Autodesk Fusion 360 part; units mm, degrees
(part 3 of 5)
  spline S77 degree 5 poles (-23.4359, 13.9427) (-23.4388, 13.9438) (-23.4499, 13.948) (-23.4693, 13.9553) (-23.4971, 13.9654) (-23.5331, 13.9784) (-23.5747, 13.9929) (-23.6165, 14.0072) (-23.6584, 14.0212) (-23.7004, 14.0348) (-23.7426, 14.0482) (-23.7849, 14.0612) (-23.8274, 14.074) (-23.87, 14.0865) (-23.9128, 14.0988) (-23.9556, 14.1108) (-23.9986, 14.1225) (-24.0417, 14.134) (-24.0849, 14.1453) (-24.1282, 14.1563) (-24.1716, 14.1671) (-24.2152, 14.1777) (-24.2588, 14.188) (-24.3025, 14.1981) (-24.3464, 14.208) (-24.3903, 14.2176) (-24.4343, 14.2271) (-24.4785, 14.2363) (-24.5227, 14.2453) (-24.567, 14.2541) (-24.6114, 14.2627) (-24.6559, 14.2711) (-24.7005, 14.2793) (-24.7451, 14.2873) (-24.7899, 14.2951) (-24.8347, 14.3027) (-24.8796, 14.3101) (-24.9246, 14.3173) (-24.9697, 14.3243) (-25.0148, 14.3311) (-25.06, 14.3377) (-25.1053, 14.3442) (-25.1507, 14.3504) (-25.1962, 14.3565) (-25.2417, 14.3624) (-25.2873, 14.3681) (-25.3329, 14.3736) (-25.3786, 14.3789) (-25.4244, 14.3841) (-25.4703, 14.3891) (-25.5162, 14.3939) (-25.5622, 14.3985) (-25.6082, 14.4029) (-25.6544, 14.4072) (-25.7005, 14.4113) (-25.7468, 14.4152) (-25.7931, 14.419) (-25.8395, 14.4226) (-25.8859, 14.426) (-25.9324, 14.4293) (-25.9789, 14.4323) (-26.0255, 14.4352) (-26.0628, 14.4374) (-26.0908, 14.439) (-26.1095, 14.44) (-26.1189, 14.4405) knots 0.13777296 0.13777296 0.13777296 0.13777296 0.13777296 0.13777296 0.14285714 0.15714286 0.17142857 0.18571429 0.2 0.21428571 0.22857143 0.24285714 0.25714286 0.27142857 0.28571429 0.3 0.31428571 0.32857143 0.34285714 0.35714286 0.37142857 0.38571429 0.4 0.41428571 0.42857143 0.44285714 0.45714286 0.47142857 0.48571429 0.5 0.51428571 0.52857143 0.54285714 0.55714286 0.57142857 0.58571429 0.6 0.61428571 0.62857143 0.64285714 0.65714286 0.67142857 0.68571429 0.7 0.71428571 0.72857143 0.74285714 0.75714286 0.77142857 0.78571429 0.8 0.81428571 0.82857143 0.84285714 0.85714286 0.87142857 0.88571429 0.9 0.91428571 0.92857143 0.94285714 0.95714286 0.97142857 0.98571429 1 1 1 1 1 1
  arc A39 (-26.1189, 14.4405) -> (-26.5772, 13.5785) centre (0, 0) ccw
  spline S78 degree 5 poles (-26.5772, 13.5785) (-26.5716, 13.571) (-26.5603, 13.5561) (-26.5433, 13.5337) (-26.5206, 13.504) (-26.4922, 13.467) (-26.4636, 13.4302) (-26.4349, 13.3934) (-26.4061, 13.3569) (-26.3772, 13.3204) (-26.3482, 13.2842) (-26.3191, 13.248) (-26.2899, 13.212) (-26.2605, 13.1762) (-26.2311, 13.1405) (-26.2015, 13.1049) (-26.1719, 13.0696) (-26.1421, 13.0343) (-26.1122, 12.9992) (-26.0822, 12.9643) (-26.0521, 12.9296) (-26.0219, 12.895) (-25.9916, 12.8605) (-25.9611, 12.8262) (-25.9306, 12.7921) (-25.8999, 12.7582) (-25.8691, 12.7244) (-25.8382, 12.6908) (-25.8072, 12.6573) (-25.7761, 12.6241) (-25.7448, 12.591) (-25.7135, 12.558) (-25.682, 12.5253) (-25.6504, 12.4927) (-25.6187, 12.4604) (-25.5868, 12.4282) (-25.5549, 12.3962) (-25.5228, 12.3644) (-25.4906, 12.3327) (-25.4583, 12.3013) (-25.4258, 12.2701) (-25.3933, 12.2391) (-25.3605, 12.2082) (-25.3277, 12.1776) (-25.2948, 12.1472) (-25.2617, 12.117) (-25.2284, 12.0871) (-25.1951, 12.0573) (-25.1616, 12.0278) (-25.1279, 11.9985) (-25.0942, 11.9695) (-25.0603, 11.9407) (-25.0262, 11.9121) (-24.992, 11.8837) (-24.9576, 11.8557) (-24.9231, 11.8279) (-24.8885, 11.8004) (-24.8537, 11.7731) (-24.8187, 11.7462) (-24.7835, 11.7196) (-24.7482, 11.6933) (-24.7172, 11.6706) (-24.6933, 11.6533) (-24.6765, 11.6412) (-24.6668, 11.6343) (-24.6642, 11.6325) knots -1 -1 -1 -1 -1 -1 -0.98571429 -0.97142857 -0.95714286 -0.94285714 -0.92857143 -0.91428571 -0.9 -0.88571429 -0.87142857 -0.85714286 -0.84285714 -0.82857143 -0.81428571 -0.8 -0.78571429 -0.77142857 -0.75714286 -0.74285714 -0.72857143 -0.71428571 -0.7 -0.68571429 -0.67142857 -0.65714286 -0.64285714 -0.62857143 -0.61428571 -0.6 -0.58571429 -0.57142857 -0.55714286 -0.54285714 -0.52857143 -0.51428571 -0.5 -0.48571429 -0.47142857 -0.45714286 -0.44285714 -0.42857143 -0.41428571 -0.4 -0.38571429 -0.37142857 -0.35714286 -0.34285714 -0.32857143 -0.31428571 -0.3 -0.28571429 -0.27142857 -0.25714286 -0.24285714 -0.22857143 -0.21428571 -0.2 -0.18571429 -0.17142857 -0.15714286 -0.14285714 -0.13777296 -0.13777296 -0.13777296 -0.13777296 -0.13777296 -0.13777296
  spline S79 degree 3 poles (-24.5985, 11.3854) (-24.5876, 11.4091) (-24.5813, 11.4346) (-24.579, 11.4866) (-24.583, 11.5126) (-24.5987, 11.5563) (-24.6084, 11.5742) (-24.633, 11.6066) (-24.6477, 11.6208) (-24.6642, 11.6325) knots 0 0 0 0 0.007813 0.007813 0.015626 0.015626 0.021719 0.021719 0.027811 0.027811 0.027811 0.027811
  arc A40 (-24.5985, 11.3854) -> (-24.9206, 10.6619) centre (0, 0) ccw
  spline S80 degree 3 poles (-25.1482, 10.5454) (-25.1228, 10.5397) (-25.0965, 10.539) (-25.0452, 10.5478) (-25.0206, 10.5572) (-24.9813, 10.5817) (-24.9658, 10.595) (-24.9394, 10.6259) (-24.9286, 10.6432) (-24.9206, 10.6619) knots 0 0 0 0 0.007813 0.007813 0.015626 0.015626 0.021719 0.021719 0.027811 0.027811 0.027811 0.027811
  spline S81 degree 5 poles (-25.1482, 10.5454) (-25.1513, 10.5461) (-25.1629, 10.5487) (-25.1831, 10.5531) (-25.212, 10.5594) (-25.2495, 10.5672) (-25.2927, 10.5758) (-25.3361, 10.5841) (-25.3795, 10.5921) (-25.423, 10.5998) (-25.4667, 10.6071) (-25.5104, 10.6141) (-25.5543, 10.6209) (-25.5982, 10.6274) (-25.6422, 10.6335) (-25.6863, 10.6395) (-25.7305, 10.6451) (-25.7748, 10.6505) (-25.8191, 10.6557) (-25.8636, 10.6606) (-25.9081, 10.6652) (-25.9526, 10.6696) (-25.9973, 10.6737) (-26.042, 10.6776) (-26.0868, 10.6813) (-26.1317, 10.6848) (-26.1766, 10.688) (-26.2216, 10.691) (-26.2666, 10.6938) (-26.3117, 10.6963) (-26.3569, 10.6987) (-26.4021, 10.7008) (-26.4474, 10.7027) (-26.4927, 10.7044) (-26.5381, 10.7059) (-26.5836, 10.7071) (-26.6291, 10.7082) (-26.6746, 10.7091) (-26.7202, 10.7098) (-26.7659, 10.7102) (-26.8116, 10.7105) (-26.8573, 10.7106) (-26.9031, 10.7105) (-26.949, 10.7101) (-26.9949, 10.7096) (-27.0408, 10.7089) (-27.0868, 10.708) (-27.1328, 10.707) (-27.1789, 10.7057) (-27.225, 10.7042) (-27.2711, 10.7026) (-27.3173, 10.7008) (-27.3635, 10.6988) (-27.4098, 10.6966) (-27.4561, 10.6942) (-27.5024, 10.6917) (-27.5488, 10.689) (-27.5952, 10.6861) (-27.6417, 10.683) (-27.6882, 10.6797) (-27.7347, 10.6763) (-27.7812, 10.6727) (-27.8185, 10.6697) (-27.8464, 10.6673) (-27.8651, 10.6658) (-27.8744, 10.6649) knots 0.13777296 0.13777296 0.13777296 0.13777296 0.13777296 0.13777296 0.14285714 0.15714286 0.17142857 0.18571429 0.2 0.21428571 0.22857143 0.24285714 0.25714286 0.27142857 0.28571429 0.3 0.31428571 0.32857143 0.34285714 0.35714286 0.37142857 0.38571429 0.4 0.41428571 0.42857143 0.44285714 0.45714286 0.47142857 0.48571429 0.5 0.51428571 0.52857143 0.54285714 0.55714286 0.57142857 0.58571429 0.6 0.61428571 0.62857143 0.64285714 0.65714286 0.67142857 0.68571429 0.7 0.71428571 0.72857143 0.74285714 0.75714286 0.77142857 0.78571429 0.8 0.81428571 0.82857143 0.84285714 0.85714286 0.87142857 0.88571429 0.9 0.91428571 0.92857143 0.94285714 0.95714286 0.97142857 0.98571429 1 1 1 1 1 1
  arc A41 (-27.8744, 10.6649) -> (-28.2083, 9.7475) centre (0, 0) ccw
  spline S82 degree 5 poles (-28.2083, 9.7475) (-28.2017, 9.7409) (-28.1884, 9.7277) (-28.1685, 9.7079) (-28.1419, 9.6816) (-28.1086, 9.649) (-28.0752, 9.6164) (-28.0416, 9.5841) (-28.008, 9.5519) (-27.9744, 9.5198) (-27.9406, 9.4879) (-27.9067, 9.4562) (-27.8728, 9.4246) (-27.8387, 9.3932) (-27.8046, 9.3619) (-27.7704, 9.3309) (-27.7361, 9.2999) (-27.7017, 9.2692) (-27.6672, 9.2386) (-27.6327, 9.2082) (-27.598, 9.178) (-27.5633, 9.1479) (-27.5285, 9.118) (-27.4935, 9.0883) (-27.4585, 9.0588) (-27.4234, 9.0294) (-27.3883, 9.0003) (-27.353, 8.9713) (-27.3176, 8.9425) (-27.2822, 8.9139) (-27.2466, 8.8854) (-27.211, 8.8572) (-27.1753, 8.8292) (-27.1394, 8.8013) (-27.1035, 8.7737) (-27.0675, 8.7462) (-27.0314, 8.719) (-26.9952, 8.6919) (-26.9589, 8.6651) (-26.9225, 8.6385) (-26.8861, 8.6121) (-26.8495, 8.5859) (-26.8128, 8.5599) (-26.776, 8.5342) (-26.7392, 8.5087) (-26.7022, 8.4834) (-26.6651, 8.4583) (-26.6279, 8.4335) (-26.5907, 8.4089) (-26.5533, 8.3846) (-26.5158, 8.3605) (-26.4782, 8.3367) (-26.4405, 8.3132) (-26.4027, 8.2899) (-26.3648, 8.2669) (-26.3267, 8.2441) (-26.2886, 8.2217) (-26.2503, 8.1996) (-26.2119, 8.1778) (-26.1734, 8.1563) (-26.1347, 8.1352) (-26.1009, 8.117) (-26.0748, 8.1032) (-26.0565, 8.0936) (-26.0459, 8.0882) (-26.0431, 8.0867) knots -1 -1 -1 -1 -1 -1 -0.98571429 -0.97142857 -0.95714286 -0.94285714 -0.92857143 -0.91428571 -0.9 -0.88571429 -0.87142857 -0.85714286 -0.84285714 -0.82857143 -0.81428571 -0.8 -0.78571429 -0.77142857 -0.75714286 -0.74285714 -0.72857143 -0.71428571 -0.7 -0.68571429 -0.67142857 -0.65714286 -0.64285714 -0.62857143 -0.61428571 -0.6 -0.58571429 -0.57142857 -0.55714286 -0.54285714 -0.52857143 -0.51428571 -0.5 -0.48571429 -0.47142857 -0.45714286 -0.44285714 -0.42857143 -0.41428571 -0.4 -0.38571429 -0.37142857 -0.35714286 -0.34285714 -0.32857143 -0.31428571 -0.3 -0.28571429 -0.27142857 -0.25714286 -0.24285714 -0.22857143 -0.21428571 -0.2 -0.18571429 -0.17142857 -0.15714286 -0.14285714 -0.13777296 -0.13777296 -0.13777296 -0.13777296 -0.13777296 -0.13777296
  spline S83 degree 3 poles (-25.9437, 7.8512) (-25.9361, 7.8761) (-25.9335, 7.9023) (-25.9385, 7.9541) (-25.946, 7.9793) (-25.9676, 8.0203) (-25.9798, 8.0367) (-26.0086, 8.0653) (-26.0251, 8.0774) (-26.0431, 8.0867) knots 0 0 0 0 0.007813 0.007813 0.015626 0.015626 0.021719 0.021719 0.027811 0.027811 0.027811 0.027811
  arc A42 (-25.9437, 7.8512) -> (-26.162, 7.0899) centre (0, 0) ccw
  spline S84 degree 3 poles (-26.3711, 6.9428) (-26.3452, 6.9407) (-26.3191, 6.9437) (-26.2694, 6.9595) (-26.2464, 6.9722) (-26.2109, 7.002) (-26.1974, 7.0174) (-26.1755, 7.0516) (-26.1673, 7.0703) (-26.162, 7.0899) knots 0 0 0 0 0.007813 0.007813 0.015626 0.015626 0.021719 0.021719 0.027811 0.027811 0.027811 0.027811
  spline S85 degree 5 poles (-26.3711, 6.9428) (-26.3742, 6.9431) (-26.3861, 6.944) (-26.4068, 6.9456) (-26.4362, 6.9478) (-26.4745, 6.9503) (-26.5185, 6.9528) (-26.5625, 6.955) (-26.6066, 6.9569) (-26.6508, 6.9584) (-26.695, 6.9596) (-26.7393, 6.9605) (-26.7837, 6.9611) (-26.8281, 6.9613) (-26.8726, 6.9613) (-26.9171, 6.9611) (-26.9616, 6.9605) (-27.0062, 6.9597) (-27.0508, 6.9586) (-27.0955, 6.9573) (-27.1402, 6.9557) (-27.185, 6.9538) (-27.2298, 6.9517) (-27.2746, 6.9494) (-27.3195, 6.9468) (-27.3644, 6.944) (-27.4093, 6.9409) (-27.4543, 6.9376) (-27.4993, 6.9341) (-27.5443, 6.9303) (-27.5893, 6.9264) (-27.6344, 6.9222) (-27.6795, 6.9178) (-27.7247, 6.9131) (-27.7698, 6.9083) (-27.815, 6.9032) (-27.8602, 6.898) (-27.9054, 6.8925) (-27.9507, 6.8868) (-27.996, 6.8809) (-28.0413, 6.8748) (-28.0866, 6.8685) (-28.1319, 6.862) (-28.1773, 6.8553) (-28.2227, 6.8484) (-28.268, 6.8414) (-28.3135, 6.8341) (-28.3589, 6.8266) (-28.4043, 6.8189) (-28.4498, 6.8111) (-28.4952, 6.803) (-28.5407, 6.7948) (-28.5862, 6.7864) (-28.6317, 6.7778) (-28.6772, 6.769) (-28.7228, 6.76) (-28.7683, 6.7509) (-28.8139, 6.7416) (-28.8594, 6.732) (-28.905, 6.7224) (-28.9506, 6.7125) (-28.9962, 6.7024) (-29.0327, 6.6943) (-29.06, 6.6881) (-29.0783, 6.6839) (-29.0874, 6.6818) knots 0.13777296 0.13777296 0.13777296 0.13777296 0.13777296 0.13777296 0.14285714 0.15714286 0.17142857 0.18571429 0.2 0.21428571 0.22857143 0.24285714 0.25714286 0.27142857 0.28571429 0.3 0.31428571 0.32857143 0.34285714 0.35714286 0.37142857 0.38571429 0.4 0.41428571 0.42857143 0.44285714 0.45714286 0.47142857 0.48571429 0.5 0.51428571 0.52857143 0.54285714 0.55714286 0.57142857 0.58571429 0.6 0.61428571 0.62857143 0.64285714 0.65714286 0.67142857 0.68571429 0.7 0.71428571 0.72857143 0.74285714 0.75714286 0.77142857 0.78571429 0.8 0.81428571 0.82857143 0.84285714 0.85714286 0.87142857 0.88571429 0.9 0.91428571 0.92857143 0.94285714 0.95714286 0.97142857 0.98571429 1 1 1 1 1 1
  arc A43 (-29.0874, 6.6818) -> (-29.2904, 5.7268) centre (0, 0) ccw
  spline S86 degree 5 poles (-29.2904, 5.7268) (-29.2829, 5.7212) (-29.268, 5.7099) (-29.2455, 5.6931) (-29.2155, 5.6708) (-29.1779, 5.6431) (-29.1403, 5.6156) (-29.1026, 5.5882) (-29.0648, 5.5609) (-29.027, 5.5339) (-28.9891, 5.507) (-28.9512, 5.4803) (-28.9132, 5.4537) (-28.8751, 5.4274) (-28.8369, 5.4012) (-28.7987, 5.3752) (-28.7605, 5.3493) (-28.7221, 5.3237) (-28.6838, 5.2982) (-28.6453, 5.2729) (-28.6068, 5.2478) (-28.5682, 5.2228) (-28.5295, 5.1981) (-28.4908, 5.1735) (-28.4521, 5.1491) (-28.4132, 5.125) (-28.3743, 5.101) (-28.3353, 5.0772) (-28.2963, 5.0536) (-28.2572, 5.0302) (-28.2181, 5.007) (-28.1789, 4.984) (-28.1396, 4.9612) (-28.1002, 4.9386) (-28.0608, 4.9162) (-28.0213, 4.894) (-27.9818, 4.8721) (-27.9422, 4.8503) (-27.9025, 4.8288) (-27.8628, 4.8075) (-27.823, 4.7865) (-27.7831, 4.7656) (-27.7432, 4.745) (-27.7032, 4.7246) (-27.6631, 4.7045) (-27.623, 4.6846) (-27.5828, 4.6649) (-27.5425, 4.6455) (-27.5022, 4.6264) (-27.4618, 4.6075) (-27.4213, 4.5889) (-27.3807, 4.5705) (-27.3401, 4.5525) (-27.2995, 4.5347) (-27.2587, 4.5171) (-27.2179, 4.4999) (-27.177, 4.483) (-27.136, 4.4665) (-27.0949, 4.4502) (-27.0538, 4.4343) (-27.0126, 4.4188) (-26.9766, 4.4055) (-26.9488, 4.3955) (-26.9293, 4.3885) (-26.9181, 4.3846) (-26.9151, 4.3835) knots -1 -1 -1 -1 -1 -1 -0.98571429 -0.97142857 -0.95714286 -0.94285714 -0.92857143 -0.91428571 -0.9 -0.88571429 -0.87142857 -0.85714286 -0.84285714 -0.82857143 -0.81428571 -0.8 -0.78571429 -0.77142857 -0.75714286 -0.74285714 -0.72857143 -0.71428571 -0.7 -0.68571429 -0.67142857 -0.65714286 -0.64285714 -0.62857143 -0.61428571 -0.6 -0.58571429 -0.57142857 -0.55714286 -0.54285714 -0.52857143 -0.51428571 -0.5 -0.48571429 -0.47142857 -0.45714286 -0.44285714 -0.42857143 -0.41428571 -0.4 -0.38571429 -0.37142857 -0.35714286 -0.34285714 -0.32857143 -0.31428571 -0.3 -0.28571429 -0.27142857 -0.25714286 -0.24285714 -0.22857143 -0.21428571 -0.2 -0.18571429 -0.17142857 -0.15714286 -0.14285714 -0.13777296 -0.13777296 -0.13777296 -0.13777296 -0.13777296 -0.13777296
  spline S87 degree 3 poles (-26.7838, 4.1641) (-26.7798, 4.1898) (-26.7809, 4.2161) (-26.793, 4.2668) (-26.804, 4.2907) (-26.8311, 4.3283) (-26.8454, 4.3428) (-26.878, 4.3672) (-26.896, 4.3768) (-26.9151, 4.3835) knots 0 0 0 0 0.007813 0.007813 0.015626 0.015626 0.021719 0.021719 0.027811 0.027811 0.027811 0.027811
  arc A44 (-26.7838, 4.1641) -> (-26.8941, 3.3798) centre (0, 0) ccw
  spline S88 degree 3 poles (-27.0807, 3.2051) (-27.0547, 3.2066) (-27.0293, 3.2132) (-26.9824, 3.2358) (-26.9613, 3.2516) (-26.9303, 3.286) (-26.9191, 3.3031) (-26.9022, 3.34) (-26.8966, 3.3597) (-26.8941, 3.3798) knots 0 0 0 0 0.007813 0.007813 0.015626 0.015626 0.021719 0.021719 0.027811 0.027811 0.027811 0.027811
  spline S89 degree 5 poles (-27.0807, 3.2051) (-27.0839, 3.2049) (-27.0958, 3.2042) (-27.1164, 3.2029) (-27.1459, 3.2009) (-27.1841, 3.1981) (-27.228, 3.1945) (-27.272, 3.1905) (-27.3159, 3.1862) (-27.3599, 3.1816) (-27.4038, 3.1766) (-27.4478, 3.1714) (-27.4918, 3.1657) (-27.5359, 3.1599) (-27.5799, 3.1537) (-27.6239, 3.1472) (-27.6679, 3.1405) (-27.712, 3.1334) (-27.756, 3.1262) (-27.8001, 3.1186) (-27.8442, 3.1108) (-27.8882, 3.1027) (-27.9323, 3.0944) (-27.9763, 3.0859) (-28.0204, 3.0771) (-28.0645, 3.068) (-28.1086, 3.0587) (-28.1526, 3.0492) (-28.1967, 3.0395) (-28.2407, 3.0295) (-28.2848, 3.0193) (-28.3289, 3.0088) (-28.3729, 2.9982) (-28.417, 2.9873) (-28.461, 2.9762) (-28.5051, 2.9649) (-28.5491, 2.9534) (-28.5931, 2.9417) (-28.6371, 2.9298) (-28.6812, 2.9177) (-28.7252, 2.9053) (-28.7692, 2.8928) (-28.8132, 2.88) (-28.8571, 2.8671) (-28.9011, 2.854) (-28.9451, 2.8406) (-28.989, 2.8271) (-29.033, 2.8134) (-29.0769, 2.7995) (-29.1208, 2.7854) (-29.1647, 2.7711) (-29.2086, 2.7566) (-29.2525, 2.7419) (-29.2964, 2.7271) (-29.3402, 2.712) (-29.3841, 2.6968) (-29.4279, 2.6814) (-29.4717, 2.6658) (-29.5155, 2.6501) (-29.5593, 2.6341) (-29.6031, 2.618) (-29.6468, 2.6017) (-29.6818, 2.5886) (-29.708, 2.5786) (-29.7255, 2.5719) (-29.7343, 2.5686) knots 0.13777296 0.13777296 0.13777296 0.13777296 0.13777296 0.13777296 0.14285714 0.15714286 0.17142857 0.18571429 0.2 0.21428571 0.22857143 0.24285714 0.25714286 0.27142857 0.28571429 0.3 0.31428571 0.32857143 0.34285714 0.35714286 0.37142857 0.38571429 0.4 0.41428571 0.42857143 0.44285714 0.45714286 0.47142857 0.48571429 0.5 0.51428571 0.52857143 0.54285714 0.55714286 0.57142857 0.58571429 0.6 0.61428571 0.62857143 0.64285714 0.65714286 0.67142857 0.68571429 0.7 0.71428571 0.72857143 0.74285714 0.75714286 0.77142857 0.78571429 0.8 0.81428571 0.82857143 0.84285714 0.85714286 0.87142857 0.88571429 0.9 0.91428571 0.92857143 0.94285714 0.95714286 0.97142857 0.98571429 1 1 1 1 1 1
  arc A45 (-29.7343, 2.5686) -> (-29.8024, 1.5946) centre (0, 0) ccw
  spline S90 degree 5 poles (-29.8024, 1.5946) (-29.7942, 1.5901) (-29.7778, 1.5811) (-29.7532, 1.5675) (-29.7204, 1.5496) (-29.6793, 1.5274) (-29.6382, 1.5054) (-29.5971, 1.4835) (-29.5559, 1.4618) (-29.5147, 1.4403) (-29.4734, 1.4189) (-29.4321, 1.3977) (-29.3908, 1.3767) (-29.3494, 1.3559) (-29.308, 1.3353) (-29.2666, 1.3148) (-29.2251, 1.2946) (-29.1835, 1.2745) (-29.142, 1.2546) (-29.1004, 1.2349) (-29.0587, 1.2154) (-29.017, 1.1961) (-28.9753, 1.1769) (-28.9336, 1.158) (-28.8918, 1.1393) (-28.85, 1.1207) (-28.8081, 1.1024) (-28.7662, 1.0842) (-28.7243, 1.0663) (-28.6823, 1.0486) (-28.6403, 1.031) (-28.5983, 1.0137) (-28.5562, 0.9966) (-28.5141, 0.9797) (-28.4719, 0.9631) (-28.4297, 0.9466) (-28.3875, 0.9304) (-28.3453, 0.9143) (-28.303, 0.8986) (-28.2607, 0.883) (-28.2183, 0.8677) (-28.176, 0.8526) (-28.1336, 0.8377) (-28.0911, 0.8231) (-28.0486, 0.8087) (-28.0061, 0.7946) (-27.9636, 0.7808) (-27.921, 0.7672) (-27.8784, 0.7538) (-27.8358, 0.7407) (-27.7931, 0.7279) (-27.7504, 0.7154) (-27.7076, 0.7032) (-27.6649, 0.6912) (-27.6221, 0.6795) (-27.5793, 0.6681) (-27.5364, 0.6571) (-27.4935, 0.6464) (-27.4506, 0.636) (-27.4076, 0.626) (-27.3647, 0.6163) (-27.3272, 0.6082) (-27.2983, 0.6021) (-27.278, 0.598) (-27.2663, 0.5956) (-27.2633, 0.595) knots -1 -1 -1 -1 -1 -1 -0.98571429 -0.97142857 -0.95714286 -0.94285714 -0.92857143 -0.91428571 -0.9 -0.88571429 -0.87142857 -0.85714286 -0.84285714 -0.82857143 -0.81428571 -0.8 -0.78571429 -0.77142857 -0.75714286 -0.74285714 -0.72857143 -0.71428571 -0.7 -0.68571429 -0.67142857 -0.65714286 -0.64285714 -0.62857143 -0.61428571 -0.6 -0.58571429 -0.57142857 -0.55714286 -0.54285714 -0.52857143 -0.51428571 -0.5 -0.48571429 -0.47142857 -0.45714286 -0.44285714 -0.42857143 -0.41428571 -0.4 -0.38571429 -0.37142857 -0.35714286 -0.34285714 -0.32857143 -0.31428571 -0.3 -0.28571429 -0.27142857 -0.25714286 -0.24285714 -0.22857143 -0.21428571 -0.2 -0.18571429 -0.17142857 -0.15714286 -0.14285714 -0.13777296 -0.13777296 -0.13777296 -0.13777296 -0.13777296 -0.13777296
  spline S91 degree 3 poles (-27.1027, 0.396) (-27.1023, 0.422) (-27.107, 0.4479) (-27.1261, 0.4964) (-27.1403, 0.5185) (-27.1724, 0.552) (-27.1886, 0.5644) (-27.2242, 0.584) (-27.2434, 0.591) (-27.2633, 0.595) knots 0 0 0 0 0.007813 0.007813 0.015626 0.015626 0.021719 0.021719 0.027811 0.027811 0.027811 0.027811
  arc A46 (-27.1027, 0.396) -> (-27.1027, -0.396) centre (0, 0) ccw
  spline S92 degree 3 poles (-27.2633, -0.595) (-27.2377, -0.5899) (-27.2134, -0.5798) (-27.1701, -0.5509) (-27.1515, -0.5324) (-27.1255, -0.4939) (-27.1168, -0.4755) (-27.1052, -0.4365) (-27.1024, -0.4163) (-27.1027, -0.396) knots 0 0 0 0 0.007813 0.007813 0.015626 0.015626 0.021719 0.021719 0.027811 0.027811 0.027811 0.027811
  spline S93 degree 5 poles (-27.2633, -0.595) (-27.2663, -0.5956) (-27.278, -0.598) (-27.2983, -0.6021) (-27.3272, -0.6082) (-27.3647, -0.6163) (-27.4076, -0.626) (-27.4506, -0.636) (-27.4935, -0.6464) (-27.5364, -0.6571) (-27.5793, -0.6681) (-27.6221, -0.6795) (-27.6649, -0.6912) (-27.7076, -0.7032) (-27.7504, -0.7154) (-27.7931, -0.7279) (-27.8358, -0.7407) (-27.8784, -0.7538) (-27.921, -0.7672) (-27.9636, -0.7808) (-28.0061, -0.7946) (-28.0486, -0.8087) (-28.0911, -0.8231) (-28.1336, -0.8377) (-28.176, -0.8526) (-28.2183, -0.8677) (-28.2607, -0.883) (-28.303, -0.8986) (-28.3453, -0.9143) (-28.3875, -0.9304) (-28.4297, -0.9466) (-28.4719, -0.9631) (-28.5141, -0.9797) (-28.5562, -0.9966) (-28.5983, -1.0137) (-28.6403, -1.031) (-28.6823, -1.0486) (-28.7243, -1.0663) (-28.7662, -1.0842) (-28.8081, -1.1024) (-28.85, -1.1207) (-28.8918, -1.1393) (-28.9336, -1.158) (-28.9753, -1.1769) (-29.017, -1.1961) (-29.0587, -1.2154) (-29.1004, -1.2349) (-29.142, -1.2546) (-29.1835, -1.2745) (-29.2251, -1.2946) (-29.2666, -1.3148) (-29.308, -1.3353) (-29.3494, -1.3559) (-29.3908, -1.3767) (-29.4321, -1.3977) (-29.4734, -1.4189) (-29.5147, -1.4403) (-29.5559, -1.4618) (-29.5971, -1.4835) (-29.6382, -1.5054) (-29.6793, -1.5274) (-29.7204, -1.5496) (-29.7532, -1.5675) (-29.7778, -1.5811) (-29.7942, -1.5901) (-29.8024, -1.5946) knots 0.13777296 0.13777296 0.13777296 0.13777296 0.13777296 0.13777296 0.14285714 0.15714286 0.17142857 0.18571429 0.2 0.21428571 0.22857143 0.24285714 0.25714286 0.27142857 0.28571429 0.3 0.31428571 0.32857143 0.34285714 0.35714286 0.37142857 0.38571429 0.4 0.41428571 0.42857143 0.44285714 0.45714286 0.47142857 0.48571429 0.5 0.51428571 0.52857143 0.54285714 0.55714286 0.57142857 0.58571429 0.6 0.61428571 0.62857143 0.64285714 0.65714286 0.67142857 0.68571429 0.7 0.71428571 0.72857143 0.74285714 0.75714286 0.77142857 0.78571429 0.8 0.81428571 0.82857143 0.84285714 0.85714286 0.87142857 0.88571429 0.9 0.91428571 0.92857143 0.94285714 0.95714286 0.97142857 0.98571429 1 1 1 1 1 1
  arc A47 (-29.8024, -1.5946) -> (-29.7343, -2.5686) centre (0, 0) ccw
  spline S94 degree 5 poles (-29.7343, -2.5686) (-29.7255, -2.5719) (-29.708, -2.5786) (-29.6818, -2.5886) (-29.6468, -2.6017) (-29.6031, -2.618) (-29.5593, -2.6341) (-29.5155, -2.6501) (-29.4717, -2.6658) (-29.4279, -2.6814) (-29.3841, -2.6968) (-29.3402, -2.712) (-29.2964, -2.7271) (-29.2525, -2.7419) (-29.2086, -2.7566) (-29.1647, -2.7711) (-29.1208, -2.7854) (-29.0769, -2.7995) (-29.033, -2.8134) (-28.989, -2.8271) (-28.9451, -2.8406) (-28.9011, -2.854) (-28.8571, -2.8671) (-28.8132, -2.88) (-28.7692, -2.8928) (-28.7252, -2.9053) (-28.6812, -2.9177) (-28.6371, -2.9298) (-28.5931, -2.9417) (-28.5491, -2.9534) (-28.5051, -2.9649) (-28.461, -2.9762) (-28.417, -2.9873) (-28.3729, -2.9982) (-28.3289, -3.0088) (-28.2848, -3.0193) (-28.2407, -3.0295) (-28.1967, -3.0395) (-28.1526, -3.0492) (-28.1086, -3.0587) (-28.0645, -3.068) (-28.0204, -3.0771) (-27.9763, -3.0859) (-27.9323, -3.0944) (-27.8882, -3.1027) (-27.8442, -3.1108) (-27.8001, -3.1186) (-27.756, -3.1262) (-27.712, -3.1334) (-27.6679, -3.1405) (-27.6239, -3.1472) (-27.5799, -3.1537) (-27.5359, -3.1599) (-27.4918, -3.1657) (-27.4478, -3.1714) (-27.4038, -3.1766) (-27.3599, -3.1816) (-27.3159, -3.1862) (-27.272, -3.1905) (-27.228, -3.1945) (-27.1841, -3.1981) (-27.1459, -3.2009) (-27.1164, -3.2029) (-27.0958, -3.2042) (-27.0839, -3.2049) (-27.0807, -3.2051) knots -1 -1 -1 -1 -1 -1 -0.98571429 -0.97142857 -0.95714286 -0.94285714 -0.92857143 -0.91428571 -0.9 -0.88571429 -0.87142857 -0.85714286 -0.84285714 -0.82857143 -0.81428571 -0.8 -0.78571429 -0.77142857 -0.75714286 -0.74285714 -0.72857143 -0.71428571 -0.7 -0.68571429 -0.67142857 -0.65714286 -0.64285714 -0.62857143 -0.61428571 -0.6 -0.58571429 -0.57142857 -0.55714286 -0.54285714 -0.52857143 -0.51428571 -0.5 -0.48571429 -0.47142857 -0.45714286 -0.44285714 -0.42857143 -0.41428571 -0.4 -0.38571429 -0.37142857 -0.35714286 -0.34285714 -0.32857143 -0.31428571 -0.3 -0.28571429 -0.27142857 -0.25714286 -0.24285714 -0.22857143 -0.21428571 -0.2 -0.18571429 -0.17142857 -0.15714286 -0.14285714 -0.13777296 -0.13777296 -0.13777296 -0.13777296 -0.13777296 -0.13777296
  spline S95 degree 3 poles (-26.8941, -3.3798) (-26.8973, -3.354) (-26.9056, -3.329) (-26.9312, -3.2837) (-26.9483, -3.2637) (-26.9847, -3.2351) (-27.0025, -3.225) (-27.0405, -3.2106) (-27.0605, -3.2063) (-27.0807, -3.2051) knots 0 0 0 0 0.007813 0.007813 0.015626 0.015626 0.021719 0.021719 0.027811 0.027811 0.027811 0.027811
  arc A48 (-26.8941, -3.3798) -> (-26.7838, -4.1641) centre (0, 0) ccw
  spline S96 degree 3 poles (-26.9151, -4.3835) (-26.8906, -4.3749) (-26.8679, -4.3615) (-26.829, -4.3269) (-26.8131, -4.3059) (-26.7928, -4.2643) (-26.7867, -4.2448) (-26.7807, -4.2046) (-26.7807, -4.1842) (-26.7838, -4.1641) knots 0 0 0 0 0.007813 0.007813 0.015626 0.015626 0.021719 0.021719 0.027811 0.027811 0.027811 0.027811
  spline S97 degree 5 poles (-26.9151, -4.3835) (-26.9181, -4.3846) (-26.9293, -4.3885) (-26.9488, -4.3955) (-26.9766, -4.4055) (-27.0126, -4.4188) (-27.0538, -4.4343) (-27.0949, -4.4502) (-27.136, -4.4665) (-27.177, -4.483) (-27.2179, -4.4999) (-27.2587, -4.5171) (-27.2995, -4.5347) (-27.3401, -4.5525) (-27.3807, -4.5705) (-27.4213, -4.5889) (-27.4618, -4.6075) (-27.5022, -4.6264) (-27.5425, -4.6455) (-27.5828, -4.6649) (-27.623, -4.6846) (-27.6631, -4.7045) (-27.7032, -4.7246) (-27.7432, -4.745) (-27.7831, -4.7656) (-27.823, -4.7865) (-27.8628, -4.8075) (-27.9025, -4.8288) (-27.9422, -4.8503) (-27.9818, -4.8721) (-28.0213, -4.894) (-28.0608, -4.9162) (-28.1002, -4.9386) (-28.1396, -4.9612) (-28.1789, -4.984) (-28.2181, -5.007) (-28.2572, -5.0302) (-28.2963, -5.0536) (-28.3353, -5.0772) (-28.3743, -5.101) (-28.4132, -5.125) (-28.4521, -5.1491) (-28.4908, -5.1735) (-28.5295, -5.1981) (-28.5682, -5.2228) (-28.6068, -5.2478) (-28.6453, -5.2729) (-28.6838, -5.2982) (-28.7221, -5.3237) (-28.7605, -5.3493) (-28.7987, -5.3752) (-28.8369, -5.4012) (-28.8751, -5.4274) (-28.9132, -5.4537) (-28.9512, -5.4803) (-28.9891, -5.507) (-29.027, -5.5339) (-29.0648, -5.5609) (-29.1026, -5.5882) (-29.1403, -5.6156) (-29.1779, -5.6431) (-29.2155, -5.6708) (-29.2455, -5.6931) (-29.268, -5.7099) (-29.2829, -5.7212) (-29.2904, -5.7268) knots 0.13777296 0.13777296 0.13777296 0.13777296 0.13777296 0.13777296 0.14285714 0.15714286 0.17142857 0.18571429 0.2 0.21428571 0.22857143 0.24285714 0.25714286 0.27142857 0.28571429 0.3 0.31428571 0.32857143 0.34285714 0.35714286 0.37142857 0.38571429 0.4 0.41428571 0.42857143 0.44285714 0.45714286 0.47142857 0.48571429 0.5 0.51428571 0.52857143 0.54285714 0.55714286 0.57142857 0.58571429 0.6 0.61428571 0.62857143 0.64285714 0.65714286 0.67142857 0.68571429 0.7 0.71428571 0.72857143 0.74285714 0.75714286 0.77142857 0.78571429 0.8 0.81428571 0.82857143 0.84285714 0.85714286 0.87142857 0.88571429 0.9 0.91428571 0.92857143 0.94285714 0.95714286 0.97142857 0.98571429 1 1 1 1 1 1
  arc A49 (-29.2904, -5.7268) -> (-29.0874, -6.6818) centre (0, 0) ccw
  spline S98 degree 5 poles (-29.0874, -6.6818) (-29.0783, -6.6839) (-29.06, -6.6881) (-29.0327, -6.6943) (-28.9962, -6.7024) (-28.9506, -6.7125) (-28.905, -6.7224) (-28.8594, -6.732) (-28.8139, -6.7416) (-28.7683, -6.7509) (-28.7228, -6.76) (-28.6772, -6.769) (-28.6317, -6.7778) (-28.5862, -6.7864) (-28.5407, -6.7948) (-28.4952, -6.803) (-28.4498, -6.8111) (-28.4043, -6.8189) (-28.3589, -6.8266) (-28.3135, -6.8341) (-28.268, -6.8414) (-28.2227, -6.8484) (-28.1773, -6.8553) (-28.1319, -6.862) (-28.0866, -6.8685) (-28.0413, -6.8748) (-27.996, -6.8809) (-27.9507, -6.8868) (-27.9054, -6.8925) (-27.8602, -6.898) (-27.815, -6.9032) (-27.7698, -6.9083) (-27.7247, -6.9131) (-27.6795, -6.9178) (-27.6344, -6.9222) (-27.5893, -6.9264) (-27.5443, -6.9303) (-27.4993, -6.9341) (-27.4543, -6.9376) (-27.4093, -6.9409) (-27.3644, -6.944) (-27.3195, -6.9468) (-27.2746, -6.9494) (-27.2298, -6.9517) (-27.185, -6.9538) (-27.1402, -6.9557) (-27.0955, -6.9573) (-27.0508, -6.9586) (-27.0062, -6.9597) (-26.9616, -6.9605) (-26.9171, -6.9611) (-26.8726, -6.9613) (-26.8281, -6.9613) (-26.7837, -6.9611) (-26.7393, -6.9605) (-26.695, -6.9596) (-26.6508, -6.9584) (-26.6066, -6.9569) (-26.5625, -6.955) (-26.5185, -6.9528) (-26.4745, -6.9503) (-26.4362, -6.9478) (-26.4068, -6.9456) (-26.3861, -6.944) (-26.3742, -6.9431) (-26.3711, -6.9428) knots -1 -1 -1 -1 -1 -1 -0.98571429 -0.97142857 -0.95714286 -0.94285714 -0.92857143 -0.91428571 -0.9 -0.88571429 -0.87142857 -0.85714286 -0.84285714 -0.82857143 -0.81428571 -0.8 -0.78571429 -0.77142857 -0.75714286 -0.74285714 -0.72857143 -0.71428571 -0.7 -0.68571429 -0.67142857 -0.65714286 -0.64285714 -0.62857143 -0.61428571 -0.6 -0.58571429 -0.57142857 -0.55714286 -0.54285714 -0.52857143 -0.51428571 -0.5 -0.48571429 -0.47142857 -0.45714286 -0.44285714 -0.42857143 -0.41428571 -0.4 -0.38571429 -0.37142857 -0.35714286 -0.34285714 -0.32857143 -0.31428571 -0.3 -0.28571429 -0.27142857 -0.25714286 -0.24285714 -0.22857143 -0.21428571 -0.2 -0.18571429 -0.17142857 -0.15714286 -0.14285714 -0.13777296 -0.13777296 -0.13777296 -0.13777296 -0.13777296 -0.13777296
  spline S99 degree 3 poles (-26.162, -7.0899) (-26.1688, -7.0647) (-26.1804, -7.0412) (-26.2121, -6.9998) (-26.2318, -6.9825) (-26.2719, -6.9591) (-26.2909, -6.9516) (-26.3305, -6.9426) (-26.3509, -6.9412) (-26.3711, -6.9428) knots 0 0 0 0 0.007813 0.007813 0.015626 0.015626 0.021719 0.021719 0.027811 0.027811 0.027811 0.027811
  arc A50 (-26.162, -7.0899) -> (-25.9437, -7.8512) centre (0, 0) ccw
  spline S100 degree 3 poles (-26.0431, -8.0867) (-26.02, -8.0747) (-25.9994, -8.0584) (-25.9657, -8.0187) (-25.9529, -7.9957) (-25.9386, -7.9516) (-25.9353, -7.9315) (-25.9349, -7.8908) (-25.9378, -7.8706) (-25.9437, -7.8512) knots 0 0 0 0 0.007813 0.007813 0.015626 0.015626 0.021719 0.021719 0.027811 0.027811 0.027811 0.027811
  spline S101 degree 5 poles (-26.0431, -8.0867) (-26.0459, -8.0882) (-26.0565, -8.0936) (-26.0748, -8.1032) (-26.1009, -8.117) (-26.1347, -8.1352) (-26.1734, -8.1563) (-26.2119, -8.1778) (-26.2503, -8.1996) (-26.2886, -8.2217) (-26.3267, -8.2441) (-26.3648, -8.2669) (-26.4027, -8.2899) (-26.4405, -8.3132) (-26.4782, -8.3367) (-26.5158, -8.3605) (-26.5533, -8.3846) (-26.5907, -8.4089) (-26.6279, -8.4335) (-26.6651, -8.4583) (-26.7022, -8.4834) (-26.7392, -8.5087) (-26.776, -8.5342) (-26.8128, -8.5599) (-26.8495, -8.5859) (-26.8861, -8.6121) (-26.9225, -8.6385) (-26.9589, -8.6651) (-26.9952, -8.6919) (-27.0314, -8.719) (-27.0675, -8.7462) (-27.1035, -8.7737) (-27.1394, -8.8013) (-27.1753, -8.8292) (-27.211, -8.8572) (-27.2466, -8.8854) (-27.2822, -8.9139) (-27.3176, -8.9425) (-27.353, -8.9713) (-27.3883, -9.0003) (-27.4234, -9.0294) (-27.4585, -9.0588) (-27.4935, -9.0883) (-27.5285, -9.118) (-27.5633, -9.1479) (-27.598, -9.178) (-27.6327, -9.2082) (-27.6672, -9.2386) (-27.7017, -9.2692) (-27.7361, -9.2999) (-27.7704, -9.3309) (-27.8046, -9.3619) (-27.8387, -9.3932) (-27.8728, -9.4246) (-27.9067, -9.4562) (-27.9406, -9.4879) (-27.9744, -9.5198) (-28.008, -9.5519) (-28.0416, -9.5841) (-28.0752, -9.6164) (-28.1086, -9.649) (-28.1419, -9.6816) (-28.1685, -9.7079) (-28.1884, -9.7277) (-28.2017, -9.7409) (-28.2083, -9.7475) knots 0.13777296 0.13777296 0.13777296 0.13777296 0.13777296 0.13777296 0.14285714 0.15714286 0.17142857 0.18571429 0.2 0.21428571 0.22857143 0.24285714 0.25714286 0.27142857 0.28571429 0.3 0.31428571 0.32857143 0.34285714 0.35714286 0.37142857 0.38571429 0.4 0.41428571 0.42857143 0.44285714 0.45714286 0.47142857 0.48571429 0.5 0.51428571 0.52857143 0.54285714 0.55714286 0.57142857 0.58571429 0.6 0.61428571 0.62857143 0.64285714 0.65714286 0.67142857 0.68571429 0.7 0.71428571 0.72857143 0.74285714 0.75714286 0.77142857 0.78571429 0.8 0.81428571 0.82857143 0.84285714 0.85714286 0.87142857 0.88571429 0.9 0.91428571 0.92857143 0.94285714 0.95714286 0.97142857 0.98571429 1 1 1 1 1 1
  arc A51 (-28.2083, -9.7475) -> (-27.8744, -10.6649) centre (0, 0) ccw
  spline S102 degree 5 poles (-27.8744, -10.6649) (-27.8651, -10.6658) (-27.8464, -10.6673) (-27.8185, -10.6697) (-27.7812, -10.6727) (-27.7347, -10.6763) (-27.6882, -10.6797) (-27.6417, -10.683) (-27.5952, -10.6861) (-27.5488, -10.689) (-27.5024, -10.6917) (-27.4561, -10.6942) (-27.4098, -10.6966) (-27.3635, -10.6988) (-27.3173, -10.7008) (-27.2711, -10.7026) (-27.225, -10.7042) (-27.1789, -10.7057) (-27.1328, -10.707) (-27.0868, -10.708) (-27.0408, -10.7089) (-26.9949, -10.7096) (-26.949, -10.7101) (-26.9031, -10.7105) (-26.8573, -10.7106) (-26.8116, -10.7105) (-26.7659, -10.7102) (-26.7202, -10.7098) (-26.6746, -10.7091) (-26.6291, -10.7082) (-26.5836, -10.7071) (-26.5381, -10.7059) (-26.4927, -10.7044) (-26.4474, -10.7027) (-26.4021, -10.7008) (-26.3569, -10.6987) (-26.3117, -10.6963) (-26.2666, -10.6938) (-26.2216, -10.691) (-26.1766, -10.688) (-26.1317, -10.6848) (-26.0868, -10.6813) (-26.042, -10.6776) (-25.9973, -10.6737) (-25.9526, -10.6696) (-25.9081, -10.6652) (-25.8636, -10.6606) (-25.8191, -10.6557) (-25.7748, -10.6505) (-25.7305, -10.6451) (-25.6863, -10.6395) (-25.6422, -10.6335) (-25.5982, -10.6274) (-25.5543, -10.6209) (-25.5104, -10.6141) (-25.4667, -10.6071) (-25.423, -10.5998) (-25.3795, -10.5921) (-25.3361, -10.5841) (-25.2927, -10.5758) (-25.2495, -10.5672) (-25.212, -10.5594) (-25.1831, -10.5531) (-25.1629, -10.5487) (-25.1513, -10.5461) (-25.1482, -10.5454) knots -1 -1 -1 -1 -1 -1 -0.98571429 -0.97142857 -0.95714286 -0.94285714 -0.92857143 -0.91428571 -0.9 -0.88571429 -0.87142857 -0.85714286 -0.84285714 -0.82857143 -0.81428571 -0.8 -0.78571429 -0.77142857 -0.75714286 -0.74285714 -0.72857143 -0.71428571 -0.7 -0.68571429 -0.67142857 -0.65714286 -0.64285714 -0.62857143 -0.61428571 -0.6 -0.58571429 -0.57142857 -0.55714286 -0.54285714 -0.52857143 -0.51428571 -0.5 -0.48571429 -0.47142857 -0.45714286 -0.44285714 -0.42857143 -0.41428571 -0.4 -0.38571429 -0.37142857 -0.35714286 -0.34285714 -0.32857143 -0.31428571 -0.3 -0.28571429 -0.27142857 -0.25714286 -0.24285714 -0.22857143 -0.21428571 -0.2 -0.18571429 -0.17142857 -0.15714286 -0.14285714 -0.13777296 -0.13777296 -0.13777296 -0.13777296 -0.13777296 -0.13777296
  spline S103 degree 3 poles (-24.9206, -10.6619) (-24.9309, -10.638) (-24.9457, -10.6163) (-24.9828, -10.5797) (-25.0048, -10.5653) (-25.0477, -10.5477) (-25.0676, -10.543) (-25.108, -10.5396) (-25.1284, -10.541) (-25.1482, -10.5454) knots 0 0 0 0 0.007813 0.007813 0.015626 0.015626 0.021719 0.021719 0.027811 0.027811 0.027811 0.027811
  arc A52 (-24.9206, -10.6619) -> (-24.5985, -11.3854) centre (0, 0) ccw
  spline S104 degree 3 poles (-24.6642, -11.6325) (-24.643, -11.6174) (-24.6249, -11.5984) (-24.5971, -11.5543) (-24.5876, -11.5298) (-24.5795, -11.4842) (-24.5791, -11.4638) (-24.5843, -11.4235) (-24.59, -11.4039) (-24.5985, -11.3854) knots 0 0 0 0 0.007813 0.007813 0.015626 0.015626 0.021719 0.021719 0.027811 0.027811 0.027811 0.027811
  spline S105 degree 5 poles (-24.6642, -11.6325) (-24.6668, -11.6343) (-24.6765, -11.6412) (-24.6933, -11.6533) (-24.7172, -11.6706) (-24.7482, -11.6933) (-24.7835, -11.7196) (-24.8187, -11.7462) (-24.8537, -11.7731) (-24.8885, -11.8004) (-24.9231, -11.8279) (-24.9576, -11.8557) (-24.992, -11.8837) (-25.0262, -11.9121) (-25.0603, -11.9407) (-25.0942, -11.9695) (-25.1279, -11.9985) (-25.1616, -12.0278) (-25.1951, -12.0573) (-25.2284, -12.0871) (-25.2617, -12.117) (-25.2948, -12.1472) (-25.3277, -12.1776) (-25.3605, -12.2082) (-25.3933, -12.2391) (-25.4258, -12.2701) (-25.4583, -12.3013) (-25.4906, -12.3327) (-25.5228, -12.3644) (-25.5549, -12.3962) (-25.5868, -12.4282) (-25.6187, -12.4604) (-25.6504, -12.4927) (-25.682, -12.5253) (-25.7135, -12.558) (-25.7448, -12.591) (-25.7761, -12.6241) (-25.8072, -12.6573) (-25.8382, -12.6908) (-25.8691, -12.7244) (-25.8999, -12.7582) (-25.9306, -12.7921) (-25.9611, -12.8262) (-25.9916, -12.8605) (-26.0219, -12.895) (-26.0521, -12.9296) (-26.0822, -12.9643) (-26.1122, -12.9992) (-26.1421, -13.0343) (-26.1719, -13.0696) (-26.2015, -13.1049) (-26.2311, -13.1405) (-26.2605, -13.1762) (-26.2899, -13.212) (-26.3191, -13.248) (-26.3482, -13.2842) (-26.3772, -13.3204) (-26.4061, -13.3569) (-26.4349, -13.3934) (-26.4636, -13.4302) (-26.4922, -13.467) (-26.5206, -13.504) (-26.5433, -13.5337) (-26.5603, -13.5561) (-26.5716, -13.571) (-26.5772, -13.5785) knots 0.13777296 0.13777296 0.13777296 0.13777296 0.13777296 0.13777296 0.14285714 0.15714286 0.17142857 0.18571429 0.2 0.21428571 0.22857143 0.24285714 0.25714286 0.27142857 0.28571429 0.3 0.31428571 0.32857143 0.34285714 0.35714286 0.37142857 0.38571429 0.4 0.41428571 0.42857143 0.44285714 0.45714286 0.47142857 0.48571429 0.5 0.51428571 0.52857143 0.54285714 0.55714286 0.57142857 0.58571429 0.6 0.61428571 0.62857143 0.64285714 0.65714286 0.67142857 0.68571429 0.7 0.71428571 0.72857143 0.74285714 0.75714286 0.77142857 0.78571429 0.8 0.81428571 0.82857143 0.84285714 0.85714286 0.87142857 0.88571429 0.9 0.91428571 0.92857143 0.94285714 0.95714286 0.97142857 0.98571429 1 1 1 1 1 1
  arc A53 (-26.5772, -13.5785) -> (-26.1189, -14.4405) centre (0, 0) ccw
  spline S106 degree 5 poles (-26.1189, -14.4405) (-26.1095, -14.44) (-26.0908, -14.439) (-26.0628, -14.4374) (-26.0255, -14.4352) (-25.9789, -14.4323) (-25.9324, -14.4293) (-25.8859, -14.426) (-25.8395, -14.4226) (-25.7931, -14.419) (-25.7468, -14.4152) (-25.7005, -14.4113) (-25.6544, -14.4072) (-25.6082, -14.4029) (-25.5622, -14.3985) (-25.5162, -14.3939) (-25.4703, -14.3891) (-25.4244, -14.3841) (-25.3786, -14.3789) (-25.3329, -14.3736) (-25.2873, -14.3681) (-25.2417, -14.3624) (-25.1962, -14.3565) (-25.1507, -14.3504) (-25.1053, -14.3442) (-25.06, -14.3377) (-25.0148, -14.3311) (-24.9697, -14.3243) (-24.9246, -14.3173) (-24.8796, -14.3101) (-24.8347, -14.3027) (-24.7899, -14.2951) (-24.7451, -14.2873) (-24.7005, -14.2793) (-24.6559, -14.2711) (-24.6114, -14.2627) (-24.567, -14.2541) (-24.5227, -14.2453) (-24.4785, -14.2363) (-24.4343, -14.2271) (-24.3903, -14.2176) (-24.3464, -14.208) (-24.3025, -14.1981) (-24.2588, -14.188) (-24.2152, -14.1777) (-24.1716, -14.1671) (-24.1282, -14.1563) (-24.0849, -14.1453) (-24.0417, -14.134) (-23.9986, -14.1225) (-23.9556, -14.1108) (-23.9128, -14.0988) (-23.87, -14.0865) (-23.8274, -14.074) (-23.7849, -14.0612) (-23.7426, -14.0482) (-23.7004, -14.0348) (-23.6584, -14.0212) (-23.6165, -14.0072) (-23.5747, -13.9929) (-23.5331, -13.9784) (-23.4971, -13.9654) (-23.4693, -13.9553) (-23.4499, -13.948) (-23.4388, -13.9438) (-23.4359, -13.9427) knots -1 -1 -1 -1 -1 -1 -0.98571429 -0.97142857 -0.95714286 -0.94285714 -0.92857143 -0.91428571 -0.9 -0.88571429 -0.87142857 -0.85714286 -0.84285714 -0.82857143 -0.81428571 -0.8 -0.78571429 -0.77142857 -0.75714286 -0.74285714 -0.72857143 -0.71428571 -0.7 -0.68571429 -0.67142857 -0.65714286 -0.64285714 -0.62857143 -0.61428571 -0.6 -0.58571429 -0.57142857 -0.55714286 -0.54285714 -0.52857143 -0.51428571 -0.5 -0.48571429 -0.47142857 -0.45714286 -0.44285714 -0.42857143 -0.41428571 -0.4 -0.38571429 -0.37142857 -0.35714286 -0.34285714 -0.32857143 -0.31428571 -0.3 -0.28571429 -0.27142857 -0.25714286 -0.24285714 -0.22857143 -0.21428571 -0.2 -0.18571429 -0.17142857 -0.15714286 -0.14285714 -0.13777296 -0.13777296 -0.13777296 -0.13777296 -0.13777296 -0.13777296
  spline S107 degree 3 poles (-23.1943, -14.0264) (-23.2077, -14.0041) (-23.2254, -13.9847) (-23.2673, -13.9537) (-23.291, -13.9424) (-23.336, -13.9311) (-23.3563, -13.9291) (-23.3969, -13.9314) (-23.4168, -13.9356) (-23.4359, -13.9427) knots 0 0 0 0 0.007813 0.007813 0.015626 0.015626 0.021719 0.021719 0.027811 0.027811 0.027811 0.027811
  arc A54 (-23.1943, -14.0264) -> (-22.7746, -14.6981) centre (0, 0) ccw
  spline S108 degree 3 poles (-22.8053, -14.9519) (-22.7863, -14.934) (-22.7711, -14.9126) (-22.7496, -14.8652) (-22.7436, -14.8395) (-22.742, -14.7932) (-22.7444, -14.7729) (-22.7552, -14.7338) (-22.7635, -14.7151) (-22.7746, -14.6981) knots 0 0 0 0 0.007813 0.007813 0.015626 0.015626 0.021719 0.021719 0.027811 0.027811 0.027811 0.027811
  spline S109 degree 5 poles (-22.8053, -14.9519) (-22.8075, -14.9541) (-22.8162, -14.9622) (-22.8312, -14.9765) (-22.8525, -14.997) (-22.8799, -15.0237) (-22.9113, -15.0547) (-22.9424, -15.086) (-22.9733, -15.1175) (-23.004, -15.1493) (-23.0345, -15.1814) (-23.0648, -15.2137) (-23.0949, -15.2463) (-23.1248, -15.2791) (-23.1545, -15.3122) (-23.1841, -15.3454) (-23.2135, -15.3789) (-23.2428, -15.4126) (-23.2718, -15.4465) (-23.3007, -15.4806) (-23.3294, -15.5149) (-23.358, -15.5494) (-23.3864, -15.5841) (-23.4147, -15.6189) (-23.4428, -15.654) (-23.4707, -15.6893) (-23.4985, -15.7247) (-23.5261, -15.7603) (-23.5536, -15.7961) (-23.581, -15.8321) (-23.6082, -15.8682) (-23.6352, -15.9045) (-23.6621, -15.941) (-23.6889, -15.9777) (-23.7155, -16.0145) (-23.742, -16.0514) (-23.7683, -16.0885) (-23.7945, -16.1258) (-23.8206, -16.1633) (-23.8465, -16.2008) (-23.8723, -16.2386) (-23.8979, -16.2765) (-23.9234, -16.3145) (-23.9488, -16.3527) (-23.974, -16.391) (-23.9991, -16.4295) (-24.0241, -16.4681) (-24.0489, -16.5069) (-24.0737, -16.5458) (-24.0982, -16.5848) (-24.1227, -16.624) (-24.147, -16.6633) (-24.1712, -16.7027) (-24.1952, -16.7423) (-24.2192, -16.782) (-24.243, -16.8218) (-24.2667, -16.8618) (-24.2902, -16.9019) (-24.3136, -16.9421) (-24.3369, -16.9825) (-24.3601, -17.023) (-24.3831, -17.0636) (-24.4015, -17.0961) (-24.4152, -17.1206) (-24.4243, -17.137) (-24.4288, -17.1452) knots 0.13777296 0.13777296 0.13777296 0.13777296 0.13777296 0.13777296 0.14285714 0.15714286 0.17142857 0.18571429 0.2 0.21428571 0.22857143 0.24285714 0.25714286 0.27142857 0.28571429 0.3 0.31428571 0.32857143 0.34285714 0.35714286 0.37142857 0.38571429 0.4 0.41428571 0.42857143 0.44285714 0.45714286 0.47142857 0.48571429 0.5 0.51428571 0.52857143 0.54285714 0.55714286 0.57142857 0.58571429 0.6 0.61428571 0.62857143 0.64285714 0.65714286 0.67142857 0.68571429 0.7 0.71428571 0.72857143 0.74285714 0.75714286 0.77142857 0.78571429 0.8 0.81428571 0.82857143 0.84285714 0.85714286 0.87142857 0.88571429 0.9 0.91428571 0.92857143 0.94285714 0.95714286 0.97142857 0.98571429 1 1 1 1 1 1
  arc A55 (-24.4288, -17.1452) -> (-23.855, -17.935) centre (0, 0) ccw
  spline S110 degree 5 poles (-23.855, -17.935) (-23.8458, -17.9332) (-23.8274, -17.9296) (-23.7999, -17.9242) (-23.7632, -17.9168) (-23.7175, -17.9074) (-23.6718, -17.8979) (-23.6262, -17.8882) (-23.5808, -17.8784) (-23.5353, -17.8684) (-23.49, -17.8582) (-23.4448, -17.8479) (-23.3996, -17.8374) (-23.3545, -17.8267) (-23.3095, -17.8159) (-23.2646, -17.8049) (-23.2198, -17.7938) (-23.1751, -17.7825) (-23.1305, -17.771) (-23.086, -17.7594) (-23.0415, -17.7475) (-22.9972, -17.7356) (-22.9529, -17.7234) (-22.9088, -17.7111) (-22.8647, -17.6986) (-22.8207, -17.6859) (-22.7769, -17.673) (-22.7331, -17.66) (-22.6895, -17.6468) (-22.6459, -17.6334) (-22.6025, -17.6198) (-22.5591, -17.606) (-22.5159, -17.5921) (-22.4728, -17.578) (-22.4298, -17.5637) (-22.3869, -17.5492) (-22.3441, -17.5345) (-22.3015, -17.5196) (-22.2589, -17.5045) (-22.2165, -17.4892) (-22.1742, -17.4737) (-22.1321, -17.458) (-22.09, -17.4422) (-22.0481, -17.4261) (-22.0063, -17.4098) (-21.9647, -17.3933) (-21.9232, -17.3765) (-21.8818, -17.3596) (-21.8406, -17.3424) (-21.7996, -17.325) (-21.7586, -17.3074) (-21.7179, -17.2896) (-21.6773, -17.2715) (-21.6368, -17.2532) (-21.5965, -17.2346) (-21.5564, -17.2158) (-21.5165, -17.1967) (-21.4767, -17.1773) (-21.4372, -17.1577) (-21.3979, -17.1377) (-21.3587, -17.1175) (-21.3248, -17.0997) (-21.2987, -17.0858) (-21.2805, -17.0759) (-21.2701, -17.0702) (-21.2673, -17.0687) knots -1 -1 -1 -1 -1 -1 -0.98571429 -0.97142857 -0.95714286 -0.94285714 -0.92857143 -0.91428571 -0.9 -0.88571429 -0.87142857 -0.85714286 -0.84285714 -0.82857143 -0.81428571 -0.8 -0.78571429 -0.77142857 -0.75714286 -0.74285714 -0.72857143 -0.71428571 -0.7 -0.68571429 -0.67142857 -0.65714286 -0.64285714 -0.62857143 -0.61428571 -0.6 -0.58571429 -0.57142857 -0.55714286 -0.54285714 -0.52857143 -0.51428571 -0.5 -0.48571429 -0.47142857 -0.45714286 -0.44285714 -0.42857143 -0.41428571 -0.4 -0.38571429 -0.37142857 -0.35714286 -0.34285714 -0.32857143 -0.31428571 -0.3 -0.28571429 -0.27142857 -0.25714286 -0.24285714 -0.22857143 -0.21428571 -0.2 -0.18571429 -0.17142857 -0.15714286 -0.14285714 -0.13777296 -0.13777296 -0.13777296 -0.13777296 -0.13777296 -0.13777296
  spline S111 degree 3 poles (-21.0164, -17.1179) (-21.0329, -17.0977) (-21.0531, -17.081) (-21.0989, -17.0561) (-21.124, -17.0482) (-21.17, -17.0432) (-21.1904, -17.0441) (-21.2303, -17.052) (-21.2495, -17.059) (-21.2673, -17.0687) knots 0 0 0 0 0.007813 0.007813 0.015626 0.015626 0.021719 0.021719 0.027811 0.027811 0.027811 0.027811
  arc A56 (-21.0164, -17.1179) -> (-20.5073, -17.7246) centre (0, 0) ccw
  spline S112 degree 3 poles (-20.5024, -17.9803) (-20.4862, -17.9599) (-20.474, -17.9366) (-20.4594, -17.8866) (-20.457, -17.8604) (-20.4619, -17.8143) (-20.4671, -17.7946) (-20.4832, -17.7573) (-20.4941, -17.74) (-20.5073, -17.7246) knots 0 0 0 0 0.007813 0.007813 0.015626 0.015626 0.021719 0.021719 0.027811 0.027811 0.027811 0.027811
  spline S113 degree 5 poles (-20.5024, -17.9803) (-20.5044, -17.9827) (-20.5118, -17.992) (-20.5247, -18.0083) (-20.5429, -18.0315) (-20.5664, -18.0618) (-20.5931, -18.0968) (-20.6195, -18.1321) (-20.6457, -18.1677) (-20.6717, -18.2034) (-20.6975, -18.2394) (-20.723, -18.2757) (-20.7482, -18.3121) (-20.7733, -18.3488) (-20.7982, -18.3856) (-20.8228, -18.4227) (-20.8473, -18.4599) (-20.8715, -18.4973) (-20.8956, -18.5349) (-20.9195, -18.5727) (-20.9432, -18.6107) (-20.9666, -18.6488) (-20.99, -18.6872) (-21.0131, -18.7256) (-21.036, -18.7643) (-21.0588, -18.8031) (-21.0814, -18.842) (-21.1038, -18.8812) (-21.126, -18.9204) (-21.1481, -18.9599) (-21.17, -18.9994) (-21.1917, -19.0391) (-21.2133, -19.079) (-21.2347, -19.119) (-21.2559, -19.1592) (-21.277, -19.1995) (-21.2979, -19.2399) (-21.3187, -19.2804) (-21.3392, -19.3211) (-21.3597, -19.362) (-21.38, -19.4029) (-21.4001, -19.444) (-21.4201, -19.4852) (-21.4399, -19.5266) (-21.4595, -19.568) (-21.479, -19.6096) (-21.4984, -19.6513) (-21.5176, -19.6932) (-21.5366, -19.7351) (-21.5556, -19.7772) (-21.5743, -19.8194) (-21.5929, -19.8617) (-21.6114, -19.9041) (-21.6297, -19.9467) (-21.6479, -19.9893) (-21.6659, -20.0321) (-21.6838, -20.075) (-21.7015, -20.118) (-21.7191, -20.1611) (-21.7366, -20.2043) (-21.7539, -20.2476) (-21.7711, -20.291) (-21.7847, -20.3258) (-21.7948, -20.352) (-21.8016, -20.3694) (-21.8049, -20.3782) knots 0.13777296 0.13777296 0.13777296 0.13777296 0.13777296 0.13777296 0.14285714 0.15714286 0.17142857 0.18571429 0.2 0.21428571 0.22857143 0.24285714 0.25714286 0.27142857 0.28571429 0.3 0.31428571 0.32857143 0.34285714 0.35714286 0.37142857 0.38571429 0.4 0.41428571 0.42857143 0.44285714 0.45714286 0.47142857 0.48571429 0.5 0.51428571 0.52857143 0.54285714 0.55714286 0.57142857 0.58571429 0.6 0.61428571 0.62857143 0.64285714 0.65714286 0.67142857 0.68571429 0.7 0.71428571 0.72857143 0.74285714 0.75714286 0.77142857 0.78571429 0.8 0.81428571 0.82857143 0.84285714 0.85714286 0.87142857 0.88571429 0.9 0.91428571 0.92857143 0.94285714 0.95714286 0.97142857 0.98571429 1 1 1 1 1 1
  arc A57 (-21.8049, -20.3782) -> (-21.1267, -21.0805) centre (0, 0) ccw
  spline S114 degree 5 poles (-21.1267, -21.0805) (-21.1179, -21.0774) (-21.1002, -21.0713) (-21.0737, -21.062) (-21.0384, -21.0496) (-20.9944, -21.034) (-20.9505, -21.0182) (-20.9068, -21.0023) (-20.8631, -20.9862) (-20.8195, -20.97) (-20.776, -20.9536) (-20.7327, -20.9371) (-20.6894, -20.9204) (-20.6462, -20.9036) (-20.6032, -20.8866) (-20.5603, -20.8695) (-20.5174, -20.8522) (-20.4747, -20.8348) (-20.4321, -20.8172) (-20.3897, -20.7995) (-20.3473, -20.7816) (-20.305, -20.7635) (-20.2629, -20.7453) (-20.2209, -20.727) (-20.179, -20.7085) (-20.1373, -20.6898) (-20.0956, -20.6709) (-20.0541, -20.652) (-20.0127, -20.6328) (-19.9714, -20.6135) (-19.9303, -20.594) (-19.8893, -20.5743) (-19.8484, -20.5545) (-19.8077, -20.5345) (-19.7671, -20.5144) (-19.7267, -20.494) (-19.6864, -20.4735) (-19.6462, -20.4528) (-19.6062, -20.432) (-19.5663, -20.4109) (-19.5266, -20.3897) (-19.487, -20.3683) (-19.4476, -20.3468) (-19.4083, -20.325) (-19.3692, -20.303) (-19.3303, -20.2809) (-19.2915, -20.2586) (-19.2529, -20.236) (-19.2145, -20.2133) (-19.1762, -20.1903) (-19.1382, -20.1672) (-19.1003, -20.1439) (-19.0626, -20.1203) (-19.0251, -20.0965) (-18.9878, -20.0725) (-18.9507, -20.0483) (-18.9138, -20.0238) (-18.8771, -19.9991) (-18.8407, -19.9742) (-18.8045, -19.949) (-18.7686, -19.9235) (-18.7374, -19.9011) (-18.7136, -19.8837) (-18.6969, -19.8714) (-18.6874, -19.8643) (-18.6848, -19.8624) knots -1 -1 -1 -1 -1 -1 -0.98571429 -0.97142857 -0.95714286 -0.94285714 -0.92857143 -0.91428571 -0.9 -0.88571429 -0.87142857 -0.85714286 -0.84285714 -0.82857143 -0.81428571 -0.8 -0.78571429 -0.77142857 -0.75714286 -0.74285714 -0.72857143 -0.71428571 -0.7 -0.68571429 -0.67142857 -0.65714286 -0.64285714 -0.62857143 -0.61428571 -0.6 -0.58571429 -0.57142857 -0.55714286 -0.54285714 -0.52857143 -0.51428571 -0.5 -0.48571429 -0.47142857 -0.45714286 -0.44285714 -0.42857143 -0.41428571 -0.4 -0.38571429 -0.37142857 -0.35714286 -0.34285714 -0.32857143 -0.31428571 -0.3 -0.28571429 -0.27142857 -0.25714286 -0.24285714 -0.22857143 -0.21428571 -0.2 -0.18571429 -0.17142857 -0.15714286 -0.14285714 -0.13777296 -0.13777296 -0.13777296 -0.13777296 -0.13777296 -0.13777296
  spline S115 degree 3 poles (-18.4295, -19.8763) (-18.4486, -19.8586) (-18.471, -19.8448) (-18.5198, -19.8265) (-18.5457, -19.8222) (-18.5921, -19.8237) (-18.6121, -19.8274) (-18.6505, -19.8407) (-18.6686, -19.8503) (-18.6848, -19.8624) knots 0 0 0 0 0.007813 0.007813 0.015626 0.015626 0.021719 0.021719 0.027811 0.027811 0.027811 0.027811
  arc A58 (-18.4295, -19.8763) -> (-17.841, -20.4062) centre (0, 0) ccw
  spline S116 degree 3 poles (-17.8005, -20.6587) (-17.7873, -20.6363) (-17.7785, -20.6115) (-17.771, -20.5599) (-17.7723, -20.5337) (-17.7835, -20.4887) (-17.7913, -20.4699) (-17.8125, -20.4352) (-17.8257, -20.4196) (-17.841, -20.4062) knots 0 0 0 0 0.007813 0.007813 0.015626 0.015626 0.021719 0.021719 0.027811 0.027811 0.027811 0.027811